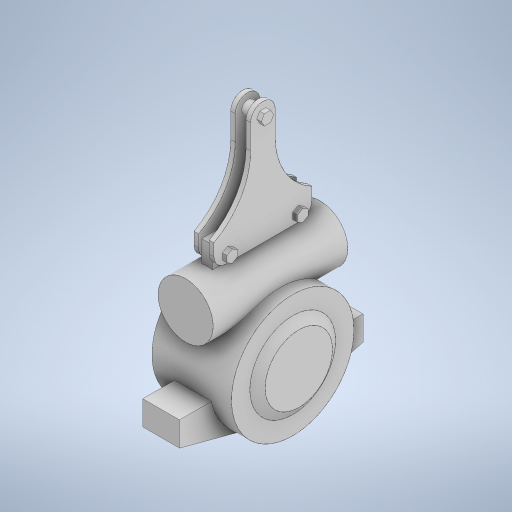
# Autodesk Inventor part: transmission_box
Saved by Autodesk Inventor 2023 (Build 270158000, 158)
## iProperties
Created: 2023-09-13
Part Number: transmission_box
Material: Generic
Document SubType Name: Modeling
Designer: Peter
Density: 1 g/cm^3
Appearance: Default
Author: Peter
Autodesk Inventor part; units mm, degrees
ref_plane "YZ Plane" through (0, 0, 0) normal (1, 0, 0) x (0, 1, 0)
ref_plane "XZ Plane" through (0, 0, 0) normal (0, 1, 0) x (-1, 0, 0)
ref_plane "XY Plane" through (0, 0, 0) normal (0, 0, 1) x (1, 0, 0)
sketch "Sketch1" plane through (0, 0, 0) normal (0, 0, 1) x (1, 0, 0)
  line L0 (-82.55, 127) -> (82.55, 127)
  line L1 (95.25, 0) -> (-82.55, 0)
  line L2 (-82.55, 0) -> (-82.55, 127)
  line L3 (82.55, 127) -> (82.55, 88.9)
  line L4 (82.55, 88.9) -> (95.25, 69.85)
  line L5 (95.25, 69.85) -> (95.25, 0)
  line L6 (0, -25.4) -> (0, 152.4) construction
  line L7 (-118.11, 0) -> (130.81, 0) construction
  point P0 (0, 127)
  dimension "d0" = 127
  dimension "d1" = 165.1
  dimension "d2" = 177.8
  dimension "d4" = 38.1
  dimension "d5" = 69.85
  dimension "d9" = 0
  constraints: 12 end point, 2 horizontal, 1 midpoint, 1 parallel, 1 perpendicular, 1 point on line, 1 vertical
  measures "d0" distance of L1.end L0.start
  measures "d1" distance of L0.start L0.end
  measures "d2" distance of L1.start L1.end
  measures "d4" distance of L0.end L3.end
  measures "d5" distance of L4.end L1.start
  measures "d9" distance between parallel lines of L7 L1
revolve "Revolution1" add sketch "Sketch1" angle 360 about axis through (95.25, 0, 0) along (-1, 0, 0)
sketch "Sketch2" plane through (0, 0, 0) normal (0, 0, 1) x (1, 0, 0)
  line L0 (82.55, 127) -> (-82.55, 127) construction
  circle A0 centre (0, 127) radius 57.15
  point P0 (0, 0)
  dimension "d6" = 114.3
  constraints: 1 centre point, 1 midpoint
  measures "d6" diameter of A0
extrude "Extrusion1" add sketch "Sketch2" along normal mid plane 279.4
sketch "Sketch3" plane through (0, 0, 0) normal (1, 0, 0) x (0, 1, 0)
  line L0 (-25.4, 190.5) -> (-25.4, -190.5)
  line L1 (-25.4, -190.5) -> (-76.2, -190.5)
  line L2 (-76.2, -190.5) -> (-127, 0)
  line L3 (-127, 0) -> (-76.2, 190.5)
  line L4 (-76.2, 190.5) -> (-25.4, 190.5)
  line L5 (-275.3083, 0) -> (260.7264, 0) construction
  line L6 (0, -293.9576) -> (0, 293.9576) construction
  line L7 (-76.2, 190.5) -> (-76.2, -190.5) construction
  point P0 (0, 0)
  point P1 (-25.4, 0)
  point P2 (-25.4, 0)
  dimension "d10" = 25.4
  dimension "d11" = 190.5
  dimension "d12" = 101.6
  dimension "d13" = 50.8
  constraints: 12 end point, 2 point on line, 2 vertical, 1 coincident, 1 midpoint, 1 parallel, 1 perpendicular
  measures "d10" distance between parallel lines of L6 L0
  measures "d11" distance between parallel lines of L1 L5
  measures "d12" distance from line of L0 L2.end
  measures "d13" distance of L0.end L1.end
extrude "Extrusion2" add sketch "Sketch3" along normal mid plane 76.2
sketch "Sketch4" plane through (0, 0, 0) normal (1, 0, 0) x (0, 1, 0)
  line L0 (228.6, 95.25) -> (133.35, 95.25)
  line L1 (133.35, 95.25) -> (133.35, 50.8)
  line L2 (133.35, 50.8) -> (228.6, 50.8)
  line L3 (228.6, 50.8) -> (228.6, 95.25)
  line L4 (184.15, -139.7) -> (184.15, 139.7) construction
  line L5 (-205.1612, 0) -> (341.967, 0) construction
  line L6 (228.6, -95.25) -> (133.35, -95.25)
  line L7 (133.35, -95.25) -> (133.35, -50.8)
  line L8 (133.35, -50.8) -> (228.6, -50.8)
  line L9 (228.6, -50.8) -> (228.6, -95.25)
  point P0 (0, 0)
  dimension "d16" = 50.8
  dimension "d17" = 44.45
  dimension "d18" = 50.8
  dimension "d19" = 44.45
  constraints: 16 end point, 4 symmetric about line, 2 parallel, 1 horizontal, 1 perpendicular
  measures "d16" distance between parallel lines of L1 L4
  measures "d17" distance between parallel lines of L3 L4
  measures "d18" distance between parallel lines of L2 L5
  measures "d19" distance of L2.end L0.start
extrude "Extrusion3" add sketch "Sketch4" along normal mid plane 22.225
sketch "Sketch5" plane through (11.1125, 0, 0) normal (1, 0, 0) x (0, 0, -1)
  line L0 (-101.6, 240.03) -> (-101.6, 214.63)
  line L1 (-76.2, 189.23) -> (76.2, 189.23)
  line L2 (101.6, 214.63) -> (101.6, 240.03)
  line L3 (-25.4, 417.83) -> (25.4, 417.83) construction
  line L4 (0, -241.046) -> (0, 557.276) construction
  line L5 (139.7, 184.15) -> (-139.7, 184.15) construction
  line L6 (-25.4, 367.03) -> (25.4, 367.03) construction
  line L7 (25.4, 367.03) -> (25.4, 417.83)
  line L8 (-25.4, 417.83) -> (-25.4, 367.03)
  arc A0 (25.4, 417.83) -> (-25.4, 417.83) centre (0, 417.83) ccw
  arc A1 (25.4, 367.03) -> (101.6, 240.03) centre (169.3333, 367.03) ccw
  arc A2 (-101.6, 240.03) -> (-25.4, 367.03) centre (-169.3333, 367.03) ccw
  line L9 (101.6, 240.03) -> (-101.6, 240.03) construction
  arc A3 (-101.6, 214.63) -> (-76.2, 189.23) centre (-76.2, 214.63) ccw
  arc A4 (76.2, 189.23) -> (101.6, 214.63) centre (76.2, 214.63) ccw
  point P0 (0, 0)
  point P1 (-101.6, 189.23)
  point P2 (101.6, 189.23)
  point P3 (0, 189.23)
  dimension "d22" = 0
  dimension "d23" = 0
  dimension "d24" = 5.08
  dimension "d25" = 50.8
  dimension "d26" = 177.8
  dimension "d27" = 50.8
  dimension "d28" = 228.6
  dimension "d29" = 203.2
  dimension "d32" = 25.4
  constraints: 16 end point, 10 point on circle, 6 tangent, 5 centre point, 4 point on line, 3 horizontal, 2 midpoint, 2 perpendicular, 2 vertical, 1 coincident, 1 equal radius, 1 parallel
  measures "d22" distance from line of L4 point (0, 189.23)
  measures "d23" distance from line of point (0, 417.83) L4
  measures "d24" distance between parallel lines of L1 L5
  measures "d25" distance of point (101.6, 189.23) L2.end
  measures "d26" distance between parallel lines of L6 L1
  measures "d27" distance of L6.start L6.end
  measures "d28" distance between parallel lines of L3 L1
  measures "d29" distance of point (-101.6, 189.23) point (101.6, 189.23)
  measures "d32" radius of A3
extrude "Extrusion4" add sketch "Sketch5" along normal blind 9.525
sketch "Sketch6" plane through (20.6375, 0, 0) normal (1, 0, 0) x (0, 0, -1)
  line L0 (-50.8, 228.6) -> (-95.25, 228.6) construction
  line L1 (0, -241.046) -> (0, 557.276) construction
  arc A0 (25.4, 417.83) -> (-25.4, 417.83) centre (0, 417.83) ccw construction
  line L2 (-12.8316, 417.83) -> (-6.4158, 428.9425)
  line L3 (-6.4158, 428.9425) -> (6.4158, 428.9425)
  line L4 (6.4158, 428.9425) -> (12.8316, 417.83)
  line L5 (12.8316, 417.83) -> (6.4158, 406.7175)
  line L6 (6.4158, 406.7175) -> (-6.4158, 406.7175)
  line L7 (-6.4158, 406.7175) -> (-12.8316, 417.83)
  line L8 (-95.25, 197.8295) -> (-95.25, 183.0592) construction
  line L9 (-73.025, 219.2066) -> (-61.9125, 212.7908)
  line L10 (-61.9125, 212.7908) -> (-61.9125, 199.9592)
  line L11 (-61.9125, 199.9592) -> (-73.025, 193.5434)
  line L12 (-73.025, 193.5434) -> (-84.1375, 199.9592)
  line L13 (-84.1375, 199.9592) -> (-84.1375, 212.7908)
  line L14 (-84.1375, 212.7908) -> (-73.025, 219.2066)
  line L15 (73.025, 219.2066) -> (61.9125, 212.7908)
  line L16 (61.9125, 212.7908) -> (61.9125, 199.9592)
  line L17 (61.9125, 199.9592) -> (73.025, 193.5434)
  line L18 (73.025, 193.5434) -> (84.1375, 199.9592)
  line L19 (84.1375, 199.9592) -> (84.1375, 212.7908)
  line L20 (84.1375, 212.7908) -> (73.025, 219.2066)
  point P0 (0, 0)
  point P1 (0, 406.7175)
  point P2 (0, 428.9425)
  point P3 (-73.025, 206.375)
  point P4 (-73.025, 228.6)
  point P5 (-73.025, 206.375)
  point P6 (-61.9125, 206.375)
  point P7 (-84.1375, 206.375)
  point P8 (73.025, 206.375)
  point P9 (95.25, 197.8295)
  point P10 (73.025, 206.375)
  point P11 (61.9125, 206.375)
  point P12 (84.1375, 206.375)
  dimension "d46" = 22.225
  dimension "d48" = 22.225
  dimension "d49" = 22.225
  dimension "d50" = 22.225
  constraints: 36 end point, 11 symmetric about line, 5 midpoint, 3 coincident, 26 other
  measures "d46" distance of point (0, 406.718) point (0, 428.942)
  measures "d48" distance from line of point (-73.025, 206.375) L8
  measures "d49" distance from line of L0 point (-73.025, 206.375)
  measures "d50" distance of point (-61.913, 206.375) point (-84.138, 206.375)
extrude "Extrusion5" add sketch "Sketch6" along normal blind 9.525
mirror "Mirror1" about plane through (0, 0, 0) normal (1, 0, 0) of "Extrusion5", "Extrusion4"
sketch "Sketch7" plane through (-11.1125, 367.03, -25.4) normal (1, 0, 0) x (0, 0, -1)
  arc A0 (0, 50.8) -> (-50.8, 50.8) centre (-25.4, 50.8) ccw construction
  circle A1 centre (-25.4, 50.8) radius 12.7
  point P0 (-25.4, -367.03)
  dimension "d43" = 25.4
  constraints: 1 centre point, 1 coincident
  measures "d43" diameter of A1
extrude "Extrusion6" add sketch "Sketch7" along normal up to next
equation "\"d48\" = d49"
body "Solid1"
